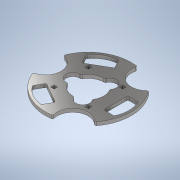
# Autodesk Inventor part: Tarcza_Tarcza_Ustalająca
Saved by Autodesk Inventor 2022 (Build 260153000, 153)
## iProperties
Created: 2021-06-13
Part Number: Tarcza_Tarcza_Ustalająca
Material: Stal, odlew
Document SubType Name: Modeling
Designer: Matik
Density: 7.85 g/cm^3
Appearance: Częściowo polerowany
Author: Matik
Autodesk Inventor part; units mm, degrees
ref_plane "YZ Plane" through (0, 0, 0) normal (1, 0, 0) x (0, 1, 0)
ref_plane "XZ Plane" through (0, 0, 0) normal (0, 1, 0) x (-1, 0, 0)
ref_plane "XY Plane" through (0, 0, 0) normal (0, 0, 1) x (1, 0, 0)
sketch "Szkic1" plane through (0, 0, 0) normal (0, 1, 0) x (-1, 0, 0)
  arc A0 (22.5, -10) -> (22.5, 10) centre (22.5, 0) ccw
  line L0 (22.5, 10) -> (21.360009, 10)
  line L1 (22.5, -10) -> (21.360009, -10)
  arc A1 (19.616335, 11.020408) -> (21.360009, 10) centre (21.360009, 12) ccw
  arc A2 (21.360009, -10) -> (19.616335, -11.020408) centre (21.360009, -12) ccw
  arc A3 (-19.352121, 11.47804) -> (-19.340259, 13.498311) centre (-21.07231, 12.498311) ccw
  line L2 (-19.910254, 14.485572) -> (-19.340259, 13.498311)
  arc A4 (-2.589746, 24.485572) -> (-19.910254, 14.485572) centre (-11.25, 19.485572) ccw
  line L3 (-2.589746, 24.485572) -> (-2.019751, 23.498311)
  arc A5 (-2.019751, 23.498311) -> (-0.264214, 22.498449) centre (-0.2877, 24.498311) ccw
  arc A6 (-0.264214, -22.498449) -> (-2.019751, -23.498311) centre (-0.2877, -24.498311) ccw
  line L4 (-2.589746, -24.485572) -> (-2.019751, -23.498311)
  arc A7 (-19.910254, -14.485572) -> (-2.589746, -24.485572) centre (-11.25, -19.485572) ccw
  line L5 (-19.910254, -14.485572) -> (-19.340259, -13.498311)
  arc A8 (-19.340259, -13.498311) -> (-19.352121, -11.47804) centre (-21.07231, -12.498311) ccw
  arc A9 (19.616335, 11.020408) -> (-0.264214, 22.498449) centre (0, 0) ccw
  arc A10 (-19.352121, 11.47804) -> (-19.352121, -11.47804) centre (0, 0) ccw
  arc A11 (-0.264214, -22.498449) -> (19.616335, -11.020408) centre (0, 0) ccw
  circle A12 centre (0, 0) radius 62.5
  circle A13 centre (0, 0) radius 40
  line L6 (-40, 0) -> (-40, 15.5)
  line L7 (-40, 0) -> (-40, -15.5)
  line L8 (-42, -17.5) -> (-53.726364, -17.5)
  line L9 (-53.726364, 17.5) -> (-42, 17.5)
  arc A14 (-55.552422, 16.315789) -> (-55.552422, -16.315789) centre (-19.031264, 0) ccw
  arc A15 (-42, -17.5) -> (-40, -15.5) centre (-42, -15.5) ccw
  arc A16 (-40, 15.5) -> (-42, 17.5) centre (-42, 15.5) ccw
  arc A17 (-53.726364, 17.5) -> (-55.552422, 16.315789) centre (-53.726364, 15.5) ccw
  arc A18 (-55.552422, -16.315789) -> (-53.726364, -17.5) centre (-53.726364, -15.5) ccw
  line L10 (20, -34.641016) -> (33.423394, -26.891016)
  arc A19 (11.707737, -55.278396) -> (13.646323, -56.267703) centre (13.439788, -54.278396) ccw
  line L11 (36.155445, -27.623067) -> (42.018627, -37.778396)
  arc A20 (13.646323, -56.267703) -> (41.906099, -39.951914) centre (9.515632, -16.481558) ccw
  arc A21 (41.906099, -39.951914) -> (42.018627, -37.778396) centre (40.286576, -38.778396) ccw
  arc A22 (36.155445, -27.623067) -> (33.423394, -26.891016) centre (34.423394, -28.623067) ccw
  arc A23 (6.576606, -42.391016) -> (5.844555, -45.123067) centre (7.576606, -44.123067) ccw
  line L12 (20, -34.641016) -> (6.576606, -42.391016)
  line L13 (11.707737, -55.278396) -> (5.844555, -45.123067)
  line L14 (20, 34.641016) -> (6.576606, 42.391016)
  arc A24 (42.018627, 37.778396) -> (41.906099, 39.951914) centre (40.286576, 38.778396) ccw
  line L15 (5.844555, 45.123067) -> (11.707737, 55.278396)
  arc A25 (41.906099, 39.951914) -> (13.646323, 56.267703) centre (9.515632, 16.481558) ccw
  arc A26 (13.646323, 56.267703) -> (11.707737, 55.278396) centre (13.439788, 54.278396) ccw
  arc A27 (5.844555, 45.123067) -> (6.576606, 42.391016) centre (7.576606, 44.123067) ccw
  arc A28 (33.423394, 26.891016) -> (36.155445, 27.623067) centre (34.423394, 28.623067) ccw
  line L16 (20, 34.641016) -> (33.423394, 26.891016)
  line L17 (42.018627, 37.778396) -> (36.155445, 27.623067)
  arc A29 (-10.057694, -61.685434) -> (-48.392306, -39.552935) centre (-31.25, -54.126588) ccw
  arc A30 (58.45, 22.132499) -> (58.45, -22.132499) centre (62.5, 0) ccw
  arc A31 (-48.392306, 39.552935) -> (-10.057694, 61.685434) centre (-31.25, 54.126588) ccw
  point P0 (20.155644, 10)
  point P1 (20.155644, -10)
  point P2 (-40, 17.5)
  point P3 (-40, -17.5)
  point P4 (-55, -17.5)
  point P5 (-55, 17.5)
  point P6 (4.844555, -43.391016)
  point P7 (35.155445, -25.891016)
  point P8 (12.344555, -56.381397)
  point P9 (42.655445, -38.881397)
  point P10 (35.155445, 25.891016)
  point P11 (4.844555, 43.391016)
  point P12 (42.655445, 38.881397)
  point P13 (12.344555, 56.381397)
  point P14 (-10.057694, 61.685434)
  point P15 (-48.392306, 39.552935)
  dimension "d8" = 80
  dimension "d1" = 20
  dimension "d2" = 2
  dimension "d5" = 360
  dimension "d7" = 125
  dimension "d9" = 17.5
  dimension "d10" = 17.5
  dimension "d11" = 15
  dimension "d13" = 40
  dimension "d14" = 2
  dimension "d17" = 360
  dimension "d21" = 45
  dimension "d24" = 360
  constraints: 69 point on circle, 36 end point, 31 centre point, 23 point on line, 11 tangent, 4 equal radius, 3 coincident, 2 vertical, 1 horizontal, 1 horizontal alignment, 1 perpendicular, 140 other
  measures "d1" diameter of A0
  measures "d2" radius of A1
  measures "d7" diameter of A12
  measures "d9" distance of L6.start point (-40, 17.5)
  measures "d10" distance of L6.start point (-40, -17.5)
  measures "d11" distance of point (-40, -17.5) point (-55, -17.5)
  measures "d13" radius of A14
  measures "d14" radius of A15
  measures "d21" diameter of A29
sketch "Szkic1 outline for Wyciągnięcie proste1" plane through (0, 0, 0) normal (0, 1, 0) x (-1, 0, 0)
  arc A0 (-10.057694, 61.685434) -> (-48.392306, 39.552935) centre (-31.25, 54.126588) cw
  arc A1 (58.45, 22.132499) -> (-10.057694, 61.685434) centre (0, 0) ccw
  arc A2 (-48.392306, 39.552935) -> (-48.392306, -39.552935) centre (0, 0) ccw
  arc A3 (58.45, -22.132499) -> (58.45, 22.132499) centre (62.5, 0) cw
  arc A4 (-48.392306, -39.552935) -> (-10.057694, -61.685434) centre (-31.25, -54.126588) cw
  arc A5 (-10.057694, -61.685434) -> (58.45, -22.132499) centre (0, 0) ccw
  line L0 (-40, 0) -> (-40, -15.5)
  line L1 (-40, 15.5) -> (-40, 0)
  arc A6 (-42, 17.5) -> (-40, 15.5) centre (-42, 15.5) cw
  line L2 (-53.726364, 17.5) -> (-42, 17.5)
  arc A7 (-55.552422, 16.315789) -> (-53.726364, 17.5) centre (-53.726364, 15.5) cw
  arc A8 (-55.552422, -16.315789) -> (-55.552422, 16.315789) centre (-19.031264, 0) cw
  arc A9 (-53.726364, -17.5) -> (-55.552422, -16.315789) centre (-53.726364, -15.5) cw
  line L3 (-42, -17.5) -> (-53.726364, -17.5)
  arc A10 (-40, -15.5) -> (-42, -17.5) centre (-42, -15.5) cw
  line L4 (20, -34.641016) -> (33.423394, -26.891016)
  line L5 (6.576606, -42.391016) -> (20, -34.641016)
  arc A11 (5.844555, -45.123067) -> (6.576606, -42.391016) centre (7.576606, -44.123067) cw
  line L6 (11.707737, -55.278396) -> (5.844555, -45.123067)
  arc A12 (13.646323, -56.267703) -> (11.707737, -55.278396) centre (13.439788, -54.278396) cw
  arc A13 (41.906099, -39.951914) -> (13.646323, -56.267703) centre (9.515632, -16.481558) cw
  arc A14 (42.018627, -37.778396) -> (41.906099, -39.951914) centre (40.286576, -38.778396) cw
  line L7 (36.155445, -27.623067) -> (42.018627, -37.778396)
  arc A15 (33.423394, -26.891016) -> (36.155445, -27.623067) centre (34.423394, -28.623067) cw
  arc A16 (21.360009, -10) -> (19.616335, -11.020408) centre (21.360009, -12) ccw
  line L8 (22.5, -10) -> (21.360009, -10)
  arc A17 (22.5, 10) -> (22.5, -10) centre (22.5, 0) cw
  line L9 (21.360009, 10) -> (22.5, 10)
  arc A18 (19.616335, 11.020408) -> (21.360009, 10) centre (21.360009, 12) ccw
  arc A19 (-0.264214, 22.498449) -> (19.616335, 11.020408) centre (0, 0) cw
  arc A20 (-2.019751, 23.498311) -> (-0.264214, 22.498449) centre (-0.2877, 24.498311) ccw
  line L10 (-2.589746, 24.485572) -> (-2.019751, 23.498311)
  arc A21 (-19.910254, 14.485572) -> (-2.589746, 24.485572) centre (-11.25, 19.485572) cw
  line L11 (-19.340259, 13.498311) -> (-19.910254, 14.485572)
  arc A22 (-19.352121, 11.47804) -> (-19.340259, 13.498311) centre (-21.07231, 12.498311) ccw
  arc A23 (-19.352121, -11.47804) -> (-19.352121, 11.47804) centre (0, 0) cw
  arc A24 (-19.340259, -13.498311) -> (-19.352121, -11.47804) centre (-21.07231, -12.498311) ccw
  line L12 (-19.910254, -14.485572) -> (-19.340259, -13.498311)
  arc A25 (-2.589746, -24.485572) -> (-19.910254, -14.485572) centre (-11.25, -19.485572) cw
  line L13 (-2.019751, -23.498311) -> (-2.589746, -24.485572)
  arc A26 (-0.264214, -22.498449) -> (-2.019751, -23.498311) centre (-0.2877, -24.498311) ccw
  arc A27 (19.616335, -11.020408) -> (-0.264214, -22.498449) centre (0, 0) cw
  line L14 (20, 34.641016) -> (6.576606, 42.391016)
  line L15 (33.423394, 26.891016) -> (20, 34.641016)
  arc A28 (36.155445, 27.623067) -> (33.423394, 26.891016) centre (34.423394, 28.623067) cw
  line L16 (42.018627, 37.778396) -> (36.155445, 27.623067)
  arc A29 (41.906099, 39.951914) -> (42.018627, 37.778396) centre (40.286576, 38.778396) cw
  arc A30 (13.646323, 56.267703) -> (41.906099, 39.951914) centre (9.515632, 16.481558) cw
  arc A31 (11.707737, 55.278396) -> (13.646323, 56.267703) centre (13.439788, 54.278396) cw
  line L17 (5.844555, 45.123067) -> (11.707737, 55.278396)
  arc A32 (6.576606, 42.391016) -> (5.844555, 45.123067) centre (7.576606, 44.123067) cw
extrude "Wyciągnięcie proste1" add sketch "Szkic1 outline for Wyciągnięcie proste1" along normal blind 5
fillet "Zaokrąglenie1" radius 2 6 edges at (48.3923, 2.5, 39.5529) (10.0577, 2.5, 61.6854) (48.3923, 2.5, -39.5529) (10.0577, 2.5, -61.6854) (-58.45, 2.5, -22.1325) (-58.45, 2.5, 22.1325)
sketch "Szkic2" plane through (0, 5, 0) normal (0, 1, 0) x (1, 0, 0)
  line L0 (25, 25) -> (-25, 25)
  line L1 (-25, 25) -> (-25, -25)
  line L2 (-25, -25) -> (25, -25)
  line L3 (25, -25) -> (25, 25)
  line L4 (25, 25) -> (-25, -25) construction
  line L5 (-25, 25) -> (25, -25) construction
  line L6 (-22.5, -27.5) -> (-27.5, -27.5)
  line L7 (-27.5, -27.5) -> (-27.5, -22.5)
  line L8 (-27.5, -22.5) -> (-22.5, -22.5)
  line L9 (-22.5, -22.5) -> (-22.5, -27.5)
  line L10 (-22.5, -27.5) -> (-27.5, -22.5) construction
  line L11 (-27.5, -27.5) -> (-22.5, -22.5) construction
  line L12 (-22.5, 27.5) -> (-27.5, 27.5)
  line L13 (-27.5, 27.5) -> (-27.5, 22.5)
  line L14 (-27.5, 22.5) -> (-22.5, 22.5)
  line L15 (-22.5, 22.5) -> (-22.5, 27.5)
  line L16 (-22.5, 27.5) -> (-27.5, 22.5) construction
  line L17 (-27.5, 27.5) -> (-22.5, 22.5) construction
  line L18 (22.5, -22.5) -> (27.5, -22.5)
  line L19 (27.5, -22.5) -> (27.5, -27.5)
  line L20 (27.5, -27.5) -> (22.5, -27.5)
  line L21 (22.5, -27.5) -> (22.5, -22.5)
  line L22 (22.5, -22.5) -> (27.5, -27.5) construction
  line L23 (27.5, -22.5) -> (22.5, -27.5) construction
  line L24 (27.5, 22.5) -> (22.5, 22.5)
  line L25 (22.5, 22.5) -> (22.5, 27.5)
  line L26 (22.5, 27.5) -> (27.5, 27.5)
  line L27 (27.5, 27.5) -> (27.5, 22.5)
  line L28 (27.5, 22.5) -> (22.5, 27.5) construction
  line L29 (22.5, 22.5) -> (27.5, 27.5) construction
  point P0 (0, 0)
  dimension "d27" = 50
  dimension "d28" = 50
  dimension "d29" = 5
  dimension "d30" = 5
  dimension "d31" = 5
  dimension "d32" = 5
  dimension "d33" = 5
  dimension "d34" = 5
  dimension "d35" = 5
  dimension "d36" = 5
  constraints: 60 end point, 10 midpoint, 10 parallel, 5 horizontal, 5 perpendicular
  measures "d27" distance of L2.end L1.end
  measures "d28" distance of L1.end L0.end
  measures "d29" distance of L7.end L8.end
  measures "d30" distance of L6.end L7.end
  measures "d31" distance of L14.end L13.end
  measures "d32" distance of L13.end L12.end
  measures "d33" distance of L19.end L20.end
  measures "d34" distance of L19.end L18.end
  measures "d35" distance of L25.end L26.end
  measures "d36" distance of L24.end L25.end
extrude "Wyciągnięcie proste2" cut sketch "Szkic2" against normal blind 10 contours L3 L24 L25 L0 | L0 L25 L26 L27 L24 L3 | L15 L14 L1 L0 | L0 L1 L14 L13 L12 L15 | L18 L19 L20 L21 L2 L3 | L3 L2 L21 L18 | L8 L9 L2 L1 | L1 L2 L9 L6 L7 L8
equation "\"d34\" = d33"
